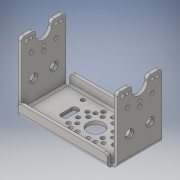
# Autodesk Inventor part: PahaAtas3D
Saved by Autodesk Inventor 2016 (Build 200138000, 138)
## iProperties
Created: 2017-02-10
Part Number: PahaAtas3D
Material: Generic
Document SubType Name: Modeling
Designer: Ghana
Density: 1 g/cm^3
Appearance: Default
Author: Ghana
Autodesk Inventor part; units mm, degrees
note: some values were not read from the file. Chosen so that the rebuilt part matches the saved one: bend side of "Bend Part14"; bend side of "Bend Part15".
ref_plane "YZ Plane" through (0, 0, 0) normal (1, 0, 0) x (0, 1, 0)
ref_plane "XZ Plane" through (0, 0, 0) normal (0, 1, 0) x (-1, 0, 0)
ref_plane "XY Plane" through (0, 0, 0) normal (0, 0, 1) x (1, 0, 0)
sketch "Sketch10" plane through (0, 0, 0) normal (0, 1, 0) x (-1, 0, 0)
  line L0 (58.159, -28) -> (58.159, 0)
  line L1 (0, -28) -> (-2, -28)
  line L2 (-2, -28) -> (-2, 0)
  line L3 (-2, 0) -> (0, 0)
  line L4 (0, 0) -> (0, -28)
  line L5 (58.159, 0) -> (94.431, 0)
  line L6 (94.431, -28) -> (58.159, -28)
  line L7 (58.159, -28) -> (58.159, 0)
  line L8 (-2, -28) -> (-38.272, -28)
  line L9 (-2, 0) -> (-2, -28)
  circle A0 centre (24.5795, -14) radius 5.2
  circle A1 centre (24.5795, -3) radius 1.25
  circle A2 centre (32.3577, -6.2218) radius 1.25
  circle A3 centre (35.5795, -14) radius 1.25
  circle A4 centre (32.3577, -21.7782) radius 1.25
  circle A5 centre (24.5795, -25) radius 1.25
  circle A6 centre (16.8013, -21.7782) radius 1.25
  circle A7 centre (13.5795, -14) radius 1.25
  circle A8 centre (16.8013, -6.2218) radius 1.25
  circle A9 centre (28.0795, -6) radius 1.35
  circle A10 centre (16.5795, -10.5) radius 1.35
  circle A11 centre (21.0795, -22) radius 1.35
  circle A12 centre (32.5795, -17.5) radius 1.35
  circle A13 centre (21.0795, -6) radius 1.25
  circle A14 centre (16.5795, -17.5) radius 1.25
  circle A15 centre (28.0795, -22) radius 1.25
  circle A16 centre (32.5795, -10.5) radius 1.25
  circle A17 centre (35.5795, -8) radius 1.35
  circle A18 centre (18.5795, -3) radius 1.35
  circle A19 centre (13.5795, -20) radius 1.35
  circle A20 centre (30.5795, -25) radius 1.35
  circle A21 centre (13.5795, -8) radius 1.25
  circle A22 centre (18.5795, -25) radius 1.25
  circle A23 centre (35.5795, -20) radius 1.25
  circle A24 centre (30.5795, -3) radius 1.25
  circle A25 centre (5.5795, -25) radius 1.25
  circle A26 centre (43.5795, -25) radius 1.25
  circle A27 centre (5.5795, -3) radius 1.25
  circle A28 centre (43.5795, -3) radius 1.25
  line L10 (40.0795, -9) -> (41.5795, -9)
  arc A29 (43.0795, -10.5) -> (41.5795, -9) centre (41.5795, -10.5) ccw
  line L11 (43.0795, -10.5) -> (43.0795, -17.5)
  arc A30 (41.5795, -19) -> (43.0795, -17.5) centre (41.5795, -17.5) ccw
  line L12 (41.5795, -19) -> (40.0795, -19)
  arc A31 (38.5795, -17.5) -> (40.0795, -19) centre (40.0795, -17.5) ccw
  line L13 (38.5795, -17.5) -> (38.5795, -10.5)
  arc A32 (40.0795, -9) -> (38.5795, -10.5) centre (40.0795, -10.5) ccw
  line L14 (10.5795, -10.5) -> (10.5795, -17.5)
  arc A33 (9.0795, -19) -> (10.5795, -17.5) centre (9.0795, -17.5) ccw
  line L15 (9.0795, -19) -> (7.5795, -19)
  arc A34 (6.0795, -17.5) -> (7.5795, -19) centre (7.5795, -17.5) ccw
  line L16 (6.0795, -17.5) -> (6.0795, -10.5)
  arc A35 (7.5795, -9) -> (6.0795, -10.5) centre (7.5795, -10.5) ccw
  line L17 (7.5795, -9) -> (9.0795, -9)
  arc A36 (10.5795, -10.5) -> (9.0795, -9) centre (9.0795, -10.5) ccw
  line L18 (93.431, -19) -> (94.431, -19)
  line L19 (93.431, -9) -> (94.431, -9)
  line L20 (96.431, -7) -> (96.431, -2)
  line L21 (96.431, -21) -> (96.431, -26)
  arc A37 (93.431, -9) -> (93.431, -19) centre (93.431, -14) ccw
  circle A38 centre (93.431, -25) radius 1.25
  circle A39 centre (93.431, -6) radius 1.0191
  circle A40 centre (85.6528, -21.7782) radius 1.25
  circle A41 centre (82.431, -14) radius 1.25
  circle A42 centre (85.6528, -6.2218) radius 1.25
  circle A43 centre (93.431, -3) radius 1.25
  circle A44 centre (85.431, -14) radius 1.0191
  circle A45 centre (93.431, -22) radius 1.0191
  arc A46 (96.431, -21) -> (94.431, -19) centre (94.431, -21) ccw
  arc A47 (94.431, -9) -> (96.431, -7) centre (94.431, -7) ccw
  arc A48 (94.431, -28) -> (96.431, -26) centre (94.431, -26) ccw
  arc A49 (96.431, -2) -> (94.431, 0) centre (94.431, -2) ccw
  line L22 (70.159, -10) -> (71.159, -10)
  line L23 (73.159, -8) -> (73.159, -7)
  line L24 (71.159, -5) -> (70.159, -5)
  line L25 (68.159, -7) -> (68.159, -8)
  arc A50 (71.159, -10) -> (73.159, -8) centre (71.159, -8) ccw
  arc A51 (68.159, -8) -> (70.159, -10) centre (70.159, -8) ccw
  arc A52 (70.159, -5) -> (68.159, -7) centre (70.159, -7) ccw
  arc A53 (73.159, -7) -> (71.159, -5) centre (71.159, -7) ccw
  line L26 (-37.272, -19) -> (-38.272, -19)
  line L27 (-37.272, -9) -> (-38.272, -9)
  line L28 (-40.272, -7) -> (-40.272, -2)
  line L29 (-40.272, -21) -> (-40.272, -26)
  arc A54 (-37.272, -19) -> (-37.272, -9) centre (-37.272, -14) ccw
  circle A55 centre (-37.272, -25) radius 1.25
  circle A56 centre (-37.272, -22) radius 1
  circle A57 centre (-29.4938, -21.7782) radius 1.25
  circle A58 centre (-26.272, -14) radius 1.25
  circle A59 centre (-29.4938, -6.2218) radius 1.25
  circle A60 centre (-37.272, -3) radius 1.25
  circle A61 centre (-29.272, -14) radius 1
  circle A62 centre (-37.272, -6) radius 1
  arc A63 (-38.272, -19) -> (-40.272, -21) centre (-38.272, -21) ccw
  arc A64 (-40.272, -7) -> (-38.272, -9) centre (-38.272, -7) ccw
  arc A65 (-40.272, -26) -> (-38.272, -28) centre (-38.272, -26) ccw
  arc A66 (-38.272, 0) -> (-40.272, -2) centre (-38.272, -2) ccw
  line L30 (-14, -10) -> (-15, -10)
  line L31 (-17, -8) -> (-17, -7)
  line L32 (-15, -5) -> (-14, -5)
  line L33 (-12, -7) -> (-12, -8)
  arc A67 (-17, -8) -> (-15, -10) centre (-15, -8) ccw
  arc A68 (-14, -10) -> (-12, -8) centre (-14, -8) ccw
  arc A69 (-12, -7) -> (-14, -5) centre (-14, -7) ccw
  arc A70 (-15, -5) -> (-17, -7) centre (-15, -7) ccw
  line L34 (-38.272, 0) -> (-2, 0)
  line L35 (70.159, -18) -> (71.159, -18)
  line L36 (73.159, -20) -> (73.159, -21)
  line L37 (71.159, -23) -> (70.159, -23)
  line L38 (68.159, -21) -> (68.159, -20)
  arc A71 (73.159, -20) -> (71.159, -18) centre (71.159, -20) ccw
  arc A72 (70.159, -18) -> (68.159, -20) centre (70.159, -20) ccw
  arc A73 (68.159, -21) -> (70.159, -23) centre (70.159, -21) ccw
  arc A74 (71.159, -23) -> (73.159, -21) centre (71.159, -21) ccw
  line L39 (-2, -14) -> (-22.3986, -14)
  line L40 (-14, -18) -> (-15, -18)
  arc A75 (-15, -18) -> (-17, -20) centre (-15, -20) ccw
  line L41 (-12, -21) -> (-12, -20)
  arc A76 (-14, -23) -> (-12, -21) centre (-14, -21) ccw
  line L42 (-17, -20) -> (-17, -21)
  line L43 (-15, -23) -> (-14, -23)
  arc A77 (-17, -21) -> (-15, -23) centre (-15, -21) ccw
  arc A78 (-12, -20) -> (-14, -18) centre (-14, -20) ccw
  line L44 (0, 0) -> (56.159, 0)
  line L45 (56.159, 0) -> (56.159, -28)
  line L46 (56.159, -28) -> (0, -28)
  line L47 (0, -28) -> (0, 0)
  line L48 (56.159, -28) -> (58.159, -28)
  line L49 (58.159, -28) -> (58.159, 0)
  line L50 (58.159, 0) -> (56.159, 0)
  line L51 (56.159, 0) -> (56.159, -28)
  line L52 (56.159, -28) -> (0, -28)
  line L53 (0, -28) -> (0, -30)
  line L54 (0, -30) -> (56.159, -30)
  line L55 (56.159, -30) -> (56.159, -28)
  line L56 (56.159, -30) -> (0, -30)
  line L57 (0, -30) -> (0, -33)
  line L58 (2, -35) -> (54.159, -35)
  line L59 (56.159, -33) -> (56.159, -30)
  line L60 (56.159, 0) -> (0, 0)
  line L61 (0, 0) -> (0, 2)
  line L62 (0, 2) -> (56.159, 2)
  line L63 (56.159, 2) -> (56.159, 0)
  line L64 (56.159, 2) -> (0, 2)
  line L65 (0, 2) -> (0, 5)
  line L66 (2, 7) -> (54.159, 7)
  line L67 (56.159, 5) -> (56.159, 2)
  arc A79 (54.159, -35) -> (56.159, -33) centre (54.159, -33) ccw
  arc A80 (0, -33) -> (2, -35) centre (2, -33) ccw
  arc A81 (56.159, 5) -> (54.159, 7) centre (54.159, 5) ccw
  arc A82 (2, 7) -> (0, 5) centre (2, 5) ccw
  point P0 (96.431, -28)
  point P1 (24.5795, -14)
  point P2 (73.159, -5)
  point P3 (73.159, -10)
  point P4 (68.159, -5)
  point P5 (-17, -5)
  point P6 (-17, -10)
  point P7 (-12, -5)
  point P8 (73.159, -23)
  point P9 (73.159, -18)
  point P10 (68.159, -23)
  point P11 (-17, -18)
  point P12 (-12, -23)
  point P13 (-17, -23)
  point P14 (0, -35)
  point P15 (56.159, -35)
  point P16 (0, 7)
  point P17 (56.159, 7)
  dimension "d81" = 2
  dimension "d87" = 38.272
  dimension "d99" = 180
  dimension "d103" = 180
  dimension "d105" = 2
  dimension "d109" = 5
  dimension "d110" = 5
  dimension "d111" = 2
  dimension "d149" = 56.159
  dimension "d150" = 2
  dimension "d151" = 56.159
  dimension "d152" = 2
  dimension "d153" = 56.159
  dimension "d154" = 5
  dimension "d155" = 56.159
  dimension "d156" = 2
  dimension "d157" = 56.159
  dimension "d158" = 5
  dimension "d159" = 2
  constraints: 136 end point, 83 centre point, 76 point on circle, 34 point on line, 24 tangent, 19 parallel, 15 symmetric about line, 11 horizontal, 9 equal radius, 9 perpendicular, 1 midpoint, 18 other
  measures "d81" distance of L3.end L2.end
  measures "d87" distance of point (96.431, -28) L0.start
  measures "d105" radius of A46
  measures "d109" distance of point (68.159, -5) point (73.159, -5)
  measures "d110" distance of point (73.159, -5) point (73.159, -10)
  measures "d111" radius of A50
  measures "d149" distance of L45.end L46.end
  measures "d150" distance of L50.end L49.end
  measures "d151" distance of L54.end L53.end
  measures "d152" distance of L53.end L52.end
  measures "d153" distance of point (56.159, -35) point (0, -35)
  measures "d154" distance of point (0, -35) L56.end
  measures "d155" distance of L61.end L62.end
  measures "d156" distance of L60.end L61.end
  measures "d157" distance of point (0, 7) point (56.159, 7)
  measures "d158" distance of L64.end point (0, 7)
  measures "d159" radius of A79
extrude "Extrusion13" add sketch "Sketch10" along normal blind 2
sketch "Sketch22" plane through (0, 2, 0) normal (0, 1, 0) x (1, 0, 0)
  circle A0 centre (-24.5795, 14) radius 5.2 projected
  arc A1 (-9.0795, 19) -> (-10.5795, 17.5) centre (-9.0795, 17.5) ccw projected
  line L0 (-9.0795, 19) -> (-7.5795, 19) projected
  arc A2 (-6.0795, 17.5) -> (-7.5795, 19) centre (-7.5795, 17.5) ccw projected
  line L1 (-6.0795, 17.5) -> (-6.0795, 10.5) projected
  arc A3 (-7.5795, 9) -> (-6.0795, 10.5) centre (-7.5795, 10.5) ccw projected
  line L2 (-7.5795, 9) -> (-9.0795, 9) projected
  arc A4 (-10.5795, 10.5) -> (-9.0795, 9) centre (-9.0795, 10.5) ccw projected
  line L3 (-10.5795, 10.5) -> (-10.5795, 17.5) projected
  arc A5 (-43.0795, 10.5) -> (-41.5795, 9) centre (-41.5795, 10.5) ccw projected
  line L4 (-43.0795, 10.5) -> (-43.0795, 17.5) projected
  arc A6 (-41.5795, 19) -> (-43.0795, 17.5) centre (-41.5795, 17.5) ccw projected
  line L5 (-41.5795, 19) -> (-40.0795, 19) projected
  arc A7 (-38.5795, 17.5) -> (-40.0795, 19) centre (-40.0795, 17.5) ccw projected
  line L6 (-38.5795, 17.5) -> (-38.5795, 10.5) projected
  arc A8 (-40.0795, 9) -> (-38.5795, 10.5) centre (-40.0795, 10.5) ccw projected
  line L7 (-40.0795, 9) -> (-41.5795, 9) projected
  circle A9 centre (-30.5795, 25) radius 1.35 projected
  circle A10 centre (-13.5795, 20) radius 1.35 projected
  circle A11 centre (-18.5795, 3) radius 1.35 projected
  circle A12 centre (-35.5795, 8) radius 1.35 projected
  circle A13 centre (-32.5795, 17.5) radius 1.35 projected
  circle A14 centre (-21.0795, 22) radius 1.35 projected
  circle A15 centre (-16.5795, 10.5) radius 1.35 projected
  circle A16 centre (-28.0795, 6) radius 1.35 projected
  circle A17 centre (-43.5795, 3) radius 1.25 projected
  circle A18 centre (-5.5795, 3) radius 1.25 projected
  circle A19 centre (-43.5795, 25) radius 1.25 projected
  circle A20 centre (-5.5795, 25) radius 1.25 projected
  circle A21 centre (-30.5795, 3) radius 1.25 projected
  circle A22 centre (-35.5795, 20) radius 1.25 projected
  circle A23 centre (-18.5795, 25) radius 1.25 projected
  circle A24 centre (-13.5795, 8) radius 1.25 projected
  circle A25 centre (-32.5795, 10.5) radius 1.25 projected
  circle A26 centre (-28.0795, 22) radius 1.25 projected
  circle A27 centre (-16.5795, 17.5) radius 1.25 projected
  circle A28 centre (-21.0795, 6) radius 1.25 projected
  circle A29 centre (-16.8013, 6.2218) radius 1.25 projected
  circle A30 centre (-13.5795, 14) radius 1.25 projected
  circle A31 centre (-16.8013, 21.7782) radius 1.25 projected
  circle A32 centre (-24.5795, 25) radius 1.25 projected
  circle A33 centre (-32.3577, 21.7782) radius 1.25 projected
  circle A34 centre (-35.5795, 14) radius 1.25 projected
  circle A35 centre (-32.3577, 6.2218) radius 1.25 projected
  circle A36 centre (-24.5795, 3) radius 1.25 projected
  arc A37 (12, 20) -> (14, 18) centre (14, 20) ccw projected
  line L8 (12, 20) -> (12, 21) projected
  arc A38 (14, 23) -> (12, 21) centre (14, 21) ccw projected
  line L9 (14, 23) -> (15, 23) projected
  arc A39 (17, 21) -> (15, 23) centre (15, 21) ccw projected
  line L10 (17, 21) -> (17, 20) projected
  arc A40 (15, 18) -> (17, 20) centre (15, 20) ccw projected
  line L11 (15, 18) -> (14, 18) projected
  arc A41 (17, 8) -> (15, 10) centre (15, 8) ccw projected
  line L12 (17, 8) -> (17, 7) projected
  arc A42 (15, 5) -> (17, 7) centre (15, 7) ccw projected
  line L13 (15, 5) -> (14, 5) projected
  arc A43 (12, 7) -> (14, 5) centre (14, 7) ccw projected
  line L14 (12, 7) -> (12, 8) projected
  arc A44 (14, 10) -> (12, 8) centre (14, 8) ccw projected
  line L15 (14, 10) -> (15, 10) projected
  circle A45 centre (37.272, 25) radius 1.25 projected
  circle A46 centre (37.272, 3) radius 1.25 projected
  circle A47 centre (29.4938, 6.2218) radius 1.25 projected
  circle A48 centre (26.272, 14) radius 1.25 projected
  circle A49 centre (29.4938, 21.7782) radius 1.25 projected
  circle A50 centre (37.272, 22) radius 1 projected
  circle A51 centre (37.272, 6) radius 1 projected
  circle A52 centre (29.272, 14) radius 1 projected
  arc A53 (-70.159, 18) -> (-68.159, 20) centre (-70.159, 20) ccw projected
  line L16 (-70.159, 18) -> (-71.159, 18) projected
  arc A54 (-73.159, 20) -> (-71.159, 18) centre (-71.159, 20) ccw projected
  line L17 (-73.159, 20) -> (-73.159, 21) projected
  arc A55 (-71.159, 23) -> (-73.159, 21) centre (-71.159, 21) ccw projected
  line L18 (-71.159, 23) -> (-70.159, 23) projected
  arc A56 (-68.159, 21) -> (-70.159, 23) centre (-70.159, 21) ccw projected
  line L19 (-68.159, 21) -> (-68.159, 20) projected
  arc A57 (-68.159, 8) -> (-70.159, 10) centre (-70.159, 8) ccw projected
  line L20 (-68.159, 8) -> (-68.159, 7) projected
  arc A58 (-70.159, 5) -> (-68.159, 7) centre (-70.159, 7) ccw projected
  line L21 (-70.159, 5) -> (-71.159, 5) projected
  arc A59 (-73.159, 7) -> (-71.159, 5) centre (-71.159, 7) ccw projected
  line L22 (-73.159, 7) -> (-73.159, 8) projected
  arc A60 (-71.159, 10) -> (-73.159, 8) centre (-71.159, 8) ccw projected
  line L23 (-71.159, 10) -> (-70.159, 10) projected
  circle A61 centre (-93.431, 3) radius 1.25 projected
  circle A62 centre (-85.6528, 6.2218) radius 1.25 projected
  circle A63 centre (-82.431, 14) radius 1.25 projected
  circle A64 centre (-85.6528, 21.7782) radius 1.25 projected
  circle A65 centre (-93.431, 25) radius 1.25 projected
  circle A66 centre (-93.431, 22) radius 1.0191 projected
  circle A67 centre (-85.431, 14) radius 1.0191 projected
  circle A68 centre (-93.431, 6) radius 1.0191 projected
  line L24 (-56.159, 28) -> (-94.431, 28) projected
  arc A69 (-94.431, 28) -> (-96.431, 26) centre (-94.431, 26) ccw projected
  line L25 (-96.431, 26) -> (-96.431, 21) projected
  arc A70 (-96.431, 21) -> (-94.431, 19) centre (-94.431, 21) ccw projected
  line L26 (-94.431, 19) -> (-93.431, 19) projected
  arc A71 (-93.431, 9) -> (-93.431, 19) centre (-93.431, 14) ccw projected
  line L27 (-93.431, 9) -> (-94.431, 9) projected
  arc A72 (-94.431, 9) -> (-96.431, 7) centre (-94.431, 7) ccw projected
  line L28 (-96.431, 7) -> (-96.431, 2) projected
  arc A73 (-96.431, 2) -> (-94.431, 0) centre (-94.431, 2) ccw projected
  line L29 (-94.431, 0) -> (-56.159, 0) projected
  line L30 (-56.159, 0) -> (-56.159, -5) projected
  arc A74 (-56.159, -5) -> (-54.159, -7) centre (-54.159, -5) ccw projected
  line L31 (-54.159, -7) -> (-2, -7) projected
  arc A75 (-2, -7) -> (0, -5) centre (-2, -5) ccw projected
  line L32 (0, -5) -> (0, 0) projected
  line L33 (0, 0) -> (38.272, 0) projected
  arc A76 (38.272, 0) -> (40.272, 2) centre (38.272, 2) ccw projected
  line L34 (40.272, 2) -> (40.272, 7) projected
  arc A77 (40.272, 7) -> (38.272, 9) centre (38.272, 7) ccw projected
  line L35 (38.272, 9) -> (37.272, 9) projected
  arc A78 (37.272, 19) -> (37.272, 9) centre (37.272, 14) ccw projected
  line L36 (37.272, 19) -> (38.272, 19) projected
  arc A79 (38.272, 19) -> (40.272, 21) centre (38.272, 21) ccw projected
  line L37 (40.272, 21) -> (40.272, 26) projected
  arc A80 (40.272, 26) -> (38.272, 28) centre (38.272, 26) ccw projected
  line L38 (38.272, 28) -> (0, 28) projected
  line L39 (0, 28) -> (0, 33) projected
  arc A81 (0, 33) -> (-2, 35) centre (-2, 33) ccw projected
  line L40 (-2, 35) -> (-54.159, 35) projected
  arc A82 (-54.159, 35) -> (-56.159, 33) centre (-54.159, 33) ccw projected
  line L41 (-56.159, 33) -> (-56.159, 28) projected
  line L42 (-94.431, 0) -> (-56.159, 0) projected
  line L43 (-56.159, 28) -> (-56.159, 0)
  constraints: 2 end point, 1 vertical
bend part "Bend Part13" radius 1.2732 angle 90 line through (-56.159, 2, -28) along (0, 0, 1) centre toward (0, 1, 0) moving side (-1, 0, 0) both sides no
sketch "Sketch23" plane through (0, 2, 0) normal (0, 1, 0) x (1, 0, 0)
  line L0 (-56.159, 0) -> (-56.159, 28) projected
  line L1 (-56.159, 0) -> (-56.159, -5) projected
  arc A0 (-56.159, -5) -> (-54.159, -7) centre (-54.159, -5) ccw projected
  line L2 (-54.159, -7) -> (-2, -7) projected
  arc A1 (-2, -7) -> (0, -5) centre (-2, -5) ccw projected
  line L3 (0, -5) -> (0, 0) projected
  line L4 (0, 0) -> (38.272, 0) projected
  arc A2 (38.272, 0) -> (40.272, 2) centre (38.272, 2) ccw projected
  line L5 (40.272, 2) -> (40.272, 7) projected
  arc A3 (40.272, 7) -> (38.272, 9) centre (38.272, 7) ccw projected
  line L6 (38.272, 9) -> (37.272, 9) projected
  arc A4 (37.272, 19) -> (37.272, 9) centre (37.272, 14) ccw projected
  line L7 (37.272, 19) -> (38.272, 19) projected
  arc A5 (38.272, 19) -> (40.272, 21) centre (38.272, 21) ccw projected
  line L8 (40.272, 21) -> (40.272, 26) projected
  arc A6 (40.272, 26) -> (38.272, 28) centre (38.272, 26) ccw projected
  line L9 (38.272, 28) -> (0, 28) projected
  line L10 (0, 28) -> (0, 33) projected
  arc A7 (0, 33) -> (-2, 35) centre (-2, 33) ccw projected
  line L11 (-2, 35) -> (-54.159, 35) projected
  arc A8 (-54.159, 35) -> (-56.159, 33) centre (-54.159, 33) ccw projected
  line L12 (-56.159, 33) -> (-56.159, 28) projected
  circle A9 centre (-24.5795, 14) radius 5.2 projected
  arc A10 (-9.0795, 19) -> (-10.5795, 17.5) centre (-9.0795, 17.5) ccw projected
  line L13 (-9.0795, 19) -> (-7.5795, 19) projected
  arc A11 (-6.0795, 17.5) -> (-7.5795, 19) centre (-7.5795, 17.5) ccw projected
  line L14 (-6.0795, 17.5) -> (-6.0795, 10.5) projected
  arc A12 (-7.5795, 9) -> (-6.0795, 10.5) centre (-7.5795, 10.5) ccw projected
  line L15 (-7.5795, 9) -> (-9.0795, 9) projected
  arc A13 (-10.5795, 10.5) -> (-9.0795, 9) centre (-9.0795, 10.5) ccw projected
  line L16 (-10.5795, 10.5) -> (-10.5795, 17.5) projected
  arc A14 (-43.0795, 10.5) -> (-41.5795, 9) centre (-41.5795, 10.5) ccw projected
  line L17 (-43.0795, 10.5) -> (-43.0795, 17.5) projected
  arc A15 (-41.5795, 19) -> (-43.0795, 17.5) centre (-41.5795, 17.5) ccw projected
  line L18 (-41.5795, 19) -> (-40.0795, 19) projected
  arc A16 (-38.5795, 17.5) -> (-40.0795, 19) centre (-40.0795, 17.5) ccw projected
  line L19 (-38.5795, 17.5) -> (-38.5795, 10.5) projected
  arc A17 (-40.0795, 9) -> (-38.5795, 10.5) centre (-40.0795, 10.5) ccw projected
  line L20 (-40.0795, 9) -> (-41.5795, 9) projected
  circle A18 centre (-30.5795, 25) radius 1.35 projected
  circle A19 centre (-13.5795, 20) radius 1.35 projected
  circle A20 centre (-18.5795, 3) radius 1.35 projected
  circle A21 centre (-35.5795, 8) radius 1.35 projected
  circle A22 centre (-32.5795, 17.5) radius 1.35 projected
  circle A23 centre (-21.0795, 22) radius 1.35 projected
  circle A24 centre (-16.5795, 10.5) radius 1.35 projected
  circle A25 centre (-28.0795, 6) radius 1.35 projected
  circle A26 centre (-43.5795, 3) radius 1.25 projected
  circle A27 centre (-5.5795, 3) radius 1.25 projected
  circle A28 centre (-43.5795, 25) radius 1.25 projected
  circle A29 centre (-5.5795, 25) radius 1.25 projected
  circle A30 centre (-30.5795, 3) radius 1.25 projected
  circle A31 centre (-35.5795, 20) radius 1.25 projected
  circle A32 centre (-18.5795, 25) radius 1.25 projected
  circle A33 centre (-13.5795, 8) radius 1.25 projected
  circle A34 centre (-32.5795, 10.5) radius 1.25 projected
  circle A35 centre (-28.0795, 22) radius 1.25 projected
  circle A36 centre (-16.5795, 17.5) radius 1.25 projected
  circle A37 centre (-21.0795, 6) radius 1.25 projected
  circle A38 centre (-16.8013, 6.2218) radius 1.25 projected
  circle A39 centre (-13.5795, 14) radius 1.25 projected
  circle A40 centre (-16.8013, 21.7782) radius 1.25 projected
  circle A41 centre (-24.5795, 25) radius 1.25 projected
  circle A42 centre (-32.3577, 21.7782) radius 1.25 projected
  circle A43 centre (-35.5795, 14) radius 1.25 projected
  circle A44 centre (-32.3577, 6.2218) radius 1.25 projected
  circle A45 centre (-24.5795, 3) radius 1.25 projected
  arc A46 (12, 20) -> (14, 18) centre (14, 20) ccw projected
  line L21 (12, 20) -> (12, 21) projected
  arc A47 (14, 23) -> (12, 21) centre (14, 21) ccw projected
  line L22 (14, 23) -> (15, 23) projected
  arc A48 (17, 21) -> (15, 23) centre (15, 21) ccw projected
  line L23 (17, 21) -> (17, 20) projected
  arc A49 (15, 18) -> (17, 20) centre (15, 20) ccw projected
  line L24 (15, 18) -> (14, 18) projected
  arc A50 (17, 8) -> (15, 10) centre (15, 8) ccw projected
  line L25 (17, 8) -> (17, 7) projected
  arc A51 (15, 5) -> (17, 7) centre (15, 7) ccw projected
  line L26 (15, 5) -> (14, 5) projected
  arc A52 (12, 7) -> (14, 5) centre (14, 7) ccw projected
  line L27 (12, 7) -> (12, 8) projected
  arc A53 (14, 10) -> (12, 8) centre (14, 8) ccw projected
  line L28 (14, 10) -> (15, 10) projected
  circle A54 centre (37.272, 25) radius 1.25 projected
  circle A55 centre (37.272, 3) radius 1.25 projected
  circle A56 centre (29.4938, 6.2218) radius 1.25 projected
  circle A57 centre (26.272, 14) radius 1.25 projected
  circle A58 centre (29.4938, 21.7782) radius 1.25 projected
  circle A59 centre (37.272, 22) radius 1 projected
  circle A60 centre (37.272, 6) radius 1 projected
  circle A61 centre (29.272, 14) radius 1 projected
  line L29 (0, 28) -> (0, 0)
  constraints: 2 end point, 1 vertical
bend part "Bend Part14" radius 1.2732 angle 90 line through (0, 2, -28) along (0, 0, 1) centre toward (0, 1, 0) moving side (1, 0, 0) both sides no
sketch "Sketch24" plane through (0, 2, 0) normal (0, 1, 0) x (1, 0, 0)
  circle A0 centre (-24.5795, 3) radius 1.25 projected
  circle A1 centre (-32.3577, 6.2218) radius 1.25 projected
  circle A2 centre (-35.5795, 14) radius 1.25 projected
  circle A3 centre (-32.3577, 21.7782) radius 1.25 projected
  circle A4 centre (-24.5795, 25) radius 1.25 projected
  circle A5 centre (-16.8013, 21.7782) radius 1.25 projected
  circle A6 centre (-13.5795, 14) radius 1.25 projected
  circle A7 centre (-16.8013, 6.2218) radius 1.25 projected
  circle A8 centre (-21.0795, 6) radius 1.25 projected
  circle A9 centre (-16.5795, 17.5) radius 1.25 projected
  circle A10 centre (-28.0795, 22) radius 1.25 projected
  circle A11 centre (-32.5795, 10.5) radius 1.25 projected
  circle A12 centre (-13.5795, 8) radius 1.25 projected
  circle A13 centre (-18.5795, 25) radius 1.25 projected
  circle A14 centre (-35.5795, 20) radius 1.25 projected
  circle A15 centre (-30.5795, 3) radius 1.25 projected
  circle A16 centre (-5.5795, 25) radius 1.25 projected
  circle A17 centre (-43.5795, 25) radius 1.25 projected
  circle A18 centre (-5.5795, 3) radius 1.25 projected
  circle A19 centre (-43.5795, 3) radius 1.25 projected
  circle A20 centre (-28.0795, 6) radius 1.35 projected
  circle A21 centre (-16.5795, 10.5) radius 1.35 projected
  circle A22 centre (-21.0795, 22) radius 1.35 projected
  circle A23 centre (-32.5795, 17.5) radius 1.35 projected
  circle A24 centre (-35.5795, 8) radius 1.35 projected
  circle A25 centre (-18.5795, 3) radius 1.35 projected
  circle A26 centre (-13.5795, 20) radius 1.35 projected
  circle A27 centre (-30.5795, 25) radius 1.35 projected
  arc A28 (-43.0795, 10.5) -> (-41.5795, 9) centre (-41.5795, 10.5) ccw projected
  line L0 (-43.0795, 10.5) -> (-43.0795, 17.5) projected
  arc A29 (-41.5795, 19) -> (-43.0795, 17.5) centre (-41.5795, 17.5) ccw projected
  line L1 (-41.5795, 19) -> (-40.0795, 19) projected
  arc A30 (-38.5795, 17.5) -> (-40.0795, 19) centre (-40.0795, 17.5) ccw projected
  line L2 (-38.5795, 17.5) -> (-38.5795, 10.5) projected
  arc A31 (-40.0795, 9) -> (-38.5795, 10.5) centre (-40.0795, 10.5) ccw projected
  line L3 (-40.0795, 9) -> (-41.5795, 9) projected
  arc A32 (-9.0795, 19) -> (-10.5795, 17.5) centre (-9.0795, 17.5) ccw projected
  line L4 (-9.0795, 19) -> (-7.5795, 19) projected
  arc A33 (-6.0795, 17.5) -> (-7.5795, 19) centre (-7.5795, 17.5) ccw projected
  line L5 (-6.0795, 17.5) -> (-6.0795, 10.5) projected
  arc A34 (-7.5795, 9) -> (-6.0795, 10.5) centre (-7.5795, 10.5) ccw projected
  line L6 (-7.5795, 9) -> (-9.0795, 9) projected
  arc A35 (-10.5795, 10.5) -> (-9.0795, 9) centre (-9.0795, 10.5) ccw projected
  line L7 (-10.5795, 10.5) -> (-10.5795, 17.5) projected
  circle A36 centre (-24.5795, 14) radius 5.2 projected
  line L8 (0, 28) -> (0, 0) projected
  line L9 (0, 28) -> (0, 33) projected
  arc A37 (0, 33) -> (-2, 35) centre (-2, 33) ccw projected
  line L10 (-2, 35) -> (-54.159, 35) projected
  arc A38 (-54.159, 35) -> (-56.159, 33) centre (-54.159, 33) ccw projected
  line L11 (-56.159, 33) -> (-56.159, 28) projected
  line L12 (-56.159, 0) -> (-56.159, 28) projected
  line L13 (-56.159, 0) -> (-56.159, -5) projected
  arc A39 (-56.159, -5) -> (-54.159, -7) centre (-54.159, -5) ccw projected
  line L14 (-54.159, -7) -> (-2, -7) projected
  arc A40 (-2, -7) -> (0, -5) centre (-2, -5) ccw projected
  line L15 (0, -5) -> (0, 0) projected
  line L16 (-56.159, 28) -> (0, 28)
  constraints: 2 end point, 1 horizontal
bend part "Bend Part15" radius 1.2732 angle 90 line through (-56.159, 2, -28) along (1, 0, 0) centre toward (0, 1, 0) moving side (0, 0, -1) both sides no
sketch "Sketch25" plane through (0, 2, 0) normal (0, 1, 0) x (1, 0, 0)
  line L0 (-56.159, 28) -> (0, 28) projected
  line L1 (-56.159, 0) -> (-56.159, 28) projected
  line L2 (-56.159, 0) -> (-56.159, -5) projected
  arc A0 (-56.159, -5) -> (-54.159, -7) centre (-54.159, -5) ccw projected
  line L3 (-54.159, -7) -> (-2, -7) projected
  arc A1 (-2, -7) -> (0, -5) centre (-2, -5) ccw projected
  line L4 (0, -5) -> (0, 0) projected
  line L5 (0, 28) -> (0, 0) projected
  circle A2 centre (-24.5795, 14) radius 5.2 projected
  arc A3 (-9.0795, 19) -> (-10.5795, 17.5) centre (-9.0795, 17.5) ccw projected
  line L6 (-9.0795, 19) -> (-7.5795, 19) projected
  arc A4 (-6.0795, 17.5) -> (-7.5795, 19) centre (-7.5795, 17.5) ccw projected
  line L7 (-6.0795, 17.5) -> (-6.0795, 10.5) projected
  arc A5 (-7.5795, 9) -> (-6.0795, 10.5) centre (-7.5795, 10.5) ccw projected
  line L8 (-7.5795, 9) -> (-9.0795, 9) projected
  arc A6 (-10.5795, 10.5) -> (-9.0795, 9) centre (-9.0795, 10.5) ccw projected
  line L9 (-10.5795, 10.5) -> (-10.5795, 17.5) projected
  arc A7 (-43.0795, 10.5) -> (-41.5795, 9) centre (-41.5795, 10.5) ccw projected
  line L10 (-43.0795, 10.5) -> (-43.0795, 17.5) projected
  arc A8 (-41.5795, 19) -> (-43.0795, 17.5) centre (-41.5795, 17.5) ccw projected
  line L11 (-41.5795, 19) -> (-40.0795, 19) projected
  arc A9 (-38.5795, 17.5) -> (-40.0795, 19) centre (-40.0795, 17.5) ccw projected
  line L12 (-38.5795, 17.5) -> (-38.5795, 10.5) projected
  arc A10 (-40.0795, 9) -> (-38.5795, 10.5) centre (-40.0795, 10.5) ccw projected
  line L13 (-40.0795, 9) -> (-41.5795, 9) projected
  circle A11 centre (-30.5795, 25) radius 1.35 projected
  circle A12 centre (-13.5795, 20) radius 1.35 projected
  circle A13 centre (-18.5795, 3) radius 1.35 projected
  circle A14 centre (-35.5795, 8) radius 1.35 projected
  circle A15 centre (-32.5795, 17.5) radius 1.35 projected
  circle A16 centre (-21.0795, 22) radius 1.35 projected
  circle A17 centre (-16.5795, 10.5) radius 1.35 projected
  circle A18 centre (-28.0795, 6) radius 1.35 projected
  circle A19 centre (-43.5795, 3) radius 1.25 projected
  circle A20 centre (-5.5795, 3) radius 1.25 projected
  circle A21 centre (-43.5795, 25) radius 1.25 projected
  circle A22 centre (-5.5795, 25) radius 1.25 projected
  circle A23 centre (-30.5795, 3) radius 1.25 projected
  circle A24 centre (-35.5795, 20) radius 1.25 projected
  circle A25 centre (-18.5795, 25) radius 1.25 projected
  circle A26 centre (-13.5795, 8) radius 1.25 projected
  circle A27 centre (-32.5795, 10.5) radius 1.25 projected
  circle A28 centre (-28.0795, 22) radius 1.25 projected
  circle A29 centre (-16.5795, 17.5) radius 1.25 projected
  circle A30 centre (-21.0795, 6) radius 1.25 projected
  circle A31 centre (-16.8013, 6.2218) radius 1.25 projected
  circle A32 centre (-13.5795, 14) radius 1.25 projected
  circle A33 centre (-16.8013, 21.7782) radius 1.25 projected
  circle A34 centre (-24.5795, 25) radius 1.25 projected
  circle A35 centre (-32.3577, 21.7782) radius 1.25 projected
  circle A36 centre (-35.5795, 14) radius 1.25 projected
  circle A37 centre (-32.3577, 6.2218) radius 1.25 projected
  circle A38 centre (-24.5795, 3) radius 1.25 projected
  line L14 (-56.159, 0) -> (0, 0)
  constraints: 2 end point, 1 horizontal
bend part "Bend Part16" radius 1.2732 angle 90 line through (-56.159, 2, 0) along (1, 0, 0) centre toward (0, 1, 0) moving side (0, 0, 1) both sides no
body "Solid4"
